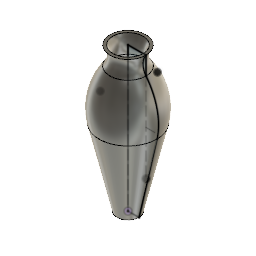
Slender_Vase (Autodesk Fusion 360 design; units mm, degrees)
Autodesk Fusion 360 part; units mm, degrees
note: some values were not read from the file. Set by a fixed rule: which sketch regions a step uses.
sketch "Sketch1" plane through (0, 0, 0) normal (0, 1, 0) x (1, 0, 0)
  line L0 (30, -240) -> (0, -240)
  line L1 (0, -240) -> (0, 0) construction
  line L2 (18.5, 0) -> (0, 0)
  line L3 (0, -240) -> (0, 0)
  line L4 (30, -240) -> (30, -210)
  line L5 (30, -210) -> (30, -61.6687) construction
  arc A0 (30, -210) -> (30, -240) centre (49.0796, -225) ccw
  line L6 (30, -135.8344) -> (50.0558, -135.8344) construction
  arc A1 (30, -210) -> (48.2433, -128.0323) centre (-46.3186, -150) ccw
  line L7 (18.5, 0) -> (48.2433, -128.0323)
  dimension "d2" = 240
  dimension "d3" = 18.5
  dimension "d4" = 30
  dimension "d32" = 30
  dimension "d34" = 148.3313
  dimension "d36" = 24.27
  dimension "d37" = 97.08
  constraint horizontal L0
  constraint vertical L1
  constraint coincident L1.end L2.end
  constraint perpendicular L1 L2
  constraint perpendicular L0 L4
  constraint parallel L4 L5
  constraint midpoint L5 L6.start
  constraint perpendicular L5 L6
  constraint tangent A1 L7
  constraint coincident L7 L6.end
  constraint tangent A0 A1
  measures "d2" distance of L1.end L0.end
  measures "d3" distance of L1.end L2.start
  measures "d4" distance of L0.start L0.end
  measures "d32" distance of L0.start L4.end
  measures "d34" distance of L4.end L5.end
  measures "d36" radius of A0
  measures "d37" radius of A1
revolve "Revolve1" add sketch "Sketch1" angle 360 about axis through (0, 0, 240) along (0, 0, -1) contours L0 L2 L3 A0 A1 L7
shell "Shell1" thickness 4 removed faces 1 at (7.6631, -11.2397, 240)
equation "d3 = ( 37 / 2 ) * 1 mm"
equation "d34 = ( 240 / 1.618 ) * 1 mm"
equation "d36 = ( 30 * ( 1.618 / 2 ) ) * 1 mm"
equation "d37 = ( 30 * ( 1.618 * 2 ) ) * 1 mm"
